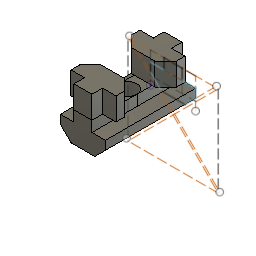
OSSM+Alux (Autodesk Fusion 360 archive; units mm, degrees)
design "4040-t-conector"
Autodesk Fusion 360 part; units mm, degrees
sketch "Sketch1" plane through (0, 0, 0) normal (0, 0, 1) x (1, 0, 0)
  line L0 (20, 0) -> (20, 13.5) construction
  line L1 (20, 13.5) -> (0, 13.5) construction
  line L2 (0, 13.5) -> (0, 0) construction
  line L3 (6, 13.5) -> (14, 13.5)
  line L4 (14, 13.5339) -> (14, 3.75) construction
  line L5 (14, 8.8) -> (6, 8.8) construction
  line L6 (6, 8.8) -> (6, 13.5) construction
  line L7 (0, 3.75) -> (20, 3.75) construction
  line L8 (-10, 13.5339) -> (30, 13.5339) construction
  line L9 (30, 13.5339) -> (30, -26.4661) construction
  line L10 (30, -26.4661) -> (-10, -26.4661) construction
  line L11 (-10, -26.4661) -> (-10, 13.5339) construction
  line L12 (-10, 13.5339) -> (30, -26.4661) construction
  line L13 (-9.2929, 14.241) -> (30.7071, -25.759) construction
  line L14 (30, 13.5339) -> (-10, -26.4661) construction
  line L15 (29.2929, 14.241) -> (-10.7071, -25.759) construction
  line L16 (0, 8.8) -> (20, 8.8) construction
  line L17 (6, 13.5) -> (6, 8.8)
  line L18 (0, 8.8) -> (0, 4.9481)
  line L19 (4.7481, 0.2) -> (15.2519, 0.2)
  line L20 (15.2519, 0.2) -> (20, 4.9481)
  line L21 (20, 4.9481) -> (20, 8.8)
  line L22 (20, 8.8) -> (14, 8.8)
  line L23 (14, 8.8) -> (14, 13.5)
  line L24 (6, 8.8) -> (0, 8.8)
  line L25 (0, 4.9481) -> (4.7481, 0.2)
  dimension "d1" = 20
  dimension "d2" = 13.5
  dimension "d3" = 8
  dimension "d4" = 4.7
  dimension "d5" = 6
  dimension "d6" = 9.75
  dimension "d7" = 40
  dimension "d8" = 40
  dimension "d9" = 10
  dimension "d10" = -1
  dimension "d11" = 1
  dimension "d21" = 13.3
  constraint vertical L0
  constraint horizontal L1
  constraint vertical L2
  constraint coincident L2.end origin
  constraint horizontal L3
  constraint vertical L4
  constraint horizontal L5
  constraint vertical L6
  constraint coincident L1 L3.start
  constraint coincident L2 L7.start
  constraint coincident L0 L7.end
  constraint perpendicular L0 L7
  constraint horizontal L8
  constraint vertical L9
  constraint horizontal L10
  constraint vertical L11
  constraint coincident L2 L16.start
  constraint coincident L0 L16.end
  constraint perpendicular L0 L16
  constraint coincident L13 L18.end
  constraint coincident L2 L18.end
  constraint coincident L13 L19.start
  constraint coincident L15 L19.end
  constraint coincident L15 L20.end
  constraint coincident L0 L20.end
  constraint coincident L7 L4.end
  constraint coincident L5.start L4
  constraint coincident L8 L4.start
  constraint coincident L3.end L4
  measures "d1" distance of L2.end L0.start
  measures "d2" distance of L2.end L1.end
  measures "d3" distance of L3.start L3.end
  measures "d4" distance of L3.start L5.end
  measures "d5" distance of L2 L6
  measures "d6" distance of L1 L7
  measures "d7" distance of L8.start L8.end
  measures "d8" distance of L8.start L10.end
  measures "d9" distance of L2 L11
  measures "d21" distance of L1 L19
extrude "Extrude1" add sketch "Sketch1" along normal blind 40 makes body 1
sketch "Sketch3" plane through (0, 0, 0) normal (0, 0, 1) x (1, 0, 0)
copy_body "CopyPasteBodies2" bodies 1 makes body 2
copy_body "CopyPasteBodies3" bodies 1 makes body 3
move_body "Move3" bodies 3 to x (1, 0, 0) y (0, 0, 1) z (0, -1, 0) at (0, 53.5, 26.5)
copy_body "CopyPasteBodies4" bodies 1 makes body 4
move_body "Move4" bodies 4 to x (1, 0, 0) y (0, 0, -1) z (0, 1, 0) at (0, 13.5, 13.5)
move_face "OffsetFaces1" offset -30 1 faces at (8.6667, 53.5, 29.5667) on bodies 3
move_face "OffsetFaces2" offset -20 1 faces at (8.6667, 53.5, 10.4333) on bodies 4
sketch "Sketch4" plane through (0, 13.5, 0) normal (0, 1, 0) x (-1, 0, 0)
  line L0 (-14, 0) -> (-6, 0)
  line L1 (-6, 0) -> (-6, 40)
  line L2 (-6, 40) -> (-14, 40)
  line L3 (-14, 40) -> (-14, 0)
  circle A0 centre (-10, 20) radius 4
  line L4 (0, 0) -> (0, 40)
  line L5 (-20, 0) -> (-20, 40)
  dimension "d16" = 8
  dimension "d17" = 20
  dimension "d18" = 10
  dimension "d22" = 20
  measures "d16" diameter of A0
  measures "d17" distance of L0 A0.centre
  measures "d18" distance of A0.centre L4
  measures "d22" distance of L4 L5
extrude "Extrude2" cut sketch "Sketch4" against normal blind 17 contours A0 bodies 1 2
combine "Combine1" operation add target body 3 tool bodies 1 4
copy_body "Body->Comp1" bodies 2 removing the originals makes body 5 in component "t-block"
move_face "OffsetFaces3" offset -10 1 faces at (8.6667, 33.5, 10.4333) on bodies 3
component "t-block" placed x (1, 0, 0) y (0, 1, 0) z (0, 0, 1) at (0, 0, 0)
equation "d5 = ( d1 - d3 ) / 2"
equation "d9 = ( d7 - d1 ) / 2"
equation "d18 = d22 / 2"
named bodies: "t-block"

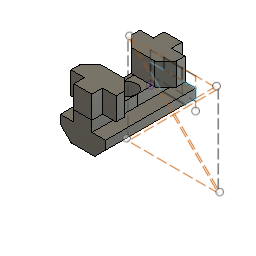
design "4040-t-conector v3"
Autodesk Fusion 360 part; units mm, degrees
sketch "Sketch1" plane through (0, 0, 0) normal (0, 0, 1) x (1, 0, 0)
  line L0 (20, 0) -> (20, 13.5) construction
  line L1 (20, 13.5) -> (0, 13.5) construction
  line L2 (0, 13.5) -> (0, 0) construction
  line L3 (6, 13.5) -> (14, 13.5)
  line L4 (14, 13.5339) -> (14, 3.75) construction
  line L5 (14, 8.8) -> (6, 8.8) construction
  line L6 (6, 8.8) -> (6, 13.5) construction
  line L7 (0, 3.75) -> (20, 3.75) construction
  line L8 (-10, 13.5339) -> (30, 13.5339) construction
  line L9 (30, 13.5339) -> (30, -26.4661) construction
  line L10 (30, -26.4661) -> (-10, -26.4661) construction
  line L11 (-10, -26.4661) -> (-10, 13.5339) construction
  line L12 (-10, 13.5339) -> (30, -26.4661) construction
  line L13 (-9.2929, 14.241) -> (30.7071, -25.759) construction
  line L14 (30, 13.5339) -> (-10, -26.4661) construction
  line L15 (29.2929, 14.241) -> (-10.7071, -25.759) construction
  line L16 (0, 8.8) -> (20, 8.8) construction
  line L17 (6, 13.5) -> (6, 8.8)
  line L18 (0, 8.8) -> (0, 4.9481)
  line L19 (4.7481, 0.2) -> (15.2519, 0.2)
  line L20 (15.2519, 0.2) -> (20, 4.9481)
  line L21 (20, 4.9481) -> (20, 8.8)
  line L22 (20, 8.8) -> (14, 8.8)
  line L23 (14, 8.8) -> (14, 13.5)
  line L24 (6, 8.8) -> (0, 8.8)
  line L25 (0, 4.9481) -> (4.7481, 0.2)
  dimension "d1" = 20
  dimension "d2" = 13.5
  dimension "d3" = 8
  dimension "d4" = 4.7
  dimension "d5" = 6
  dimension "d6" = 9.75
  dimension "d7" = 40
  dimension "d8" = 40
  dimension "d9" = 10
  dimension "d10" = -1
  dimension "d11" = 1
  dimension "d21" = 13.3
  constraint vertical L0
  constraint horizontal L1
  constraint vertical L2
  constraint coincident L2.end origin
  constraint horizontal L3
  constraint vertical L4
  constraint horizontal L5
  constraint vertical L6
  constraint coincident L1 L3.start
  constraint coincident L2 L7.start
  constraint coincident L0 L7.end
  constraint perpendicular L0 L7
  constraint horizontal L8
  constraint vertical L9
  constraint horizontal L10
  constraint vertical L11
  constraint coincident L2 L16.start
  constraint coincident L0 L16.end
  constraint perpendicular L0 L16
  constraint coincident L13 L18.end
  constraint coincident L2 L18.end
  constraint coincident L13 L19.start
  constraint coincident L15 L19.end
  constraint coincident L15 L20.end
  constraint coincident L0 L20.end
  constraint coincident L7 L4.end
  constraint coincident L5.start L4
  constraint coincident L8 L4.start
  constraint coincident L3.end L4
  measures "d1" distance of L2.end L0.start
  measures "d2" distance of L2.end L1.end
  measures "d3" distance of L3.start L3.end
  measures "d4" distance of L3.start L5.end
  measures "d5" distance of L2 L6
  measures "d6" distance of L1 L7
  measures "d7" distance of L8.start L8.end
  measures "d8" distance of L8.start L10.end
  measures "d9" distance of L2 L11
  measures "d21" distance of L1 L19
extrude "Extrude1" add sketch "Sketch1" along normal blind 40 makes body 1
sketch "Sketch3" plane through (0, 0, 0) normal (0, 0, 1) x (1, 0, 0)
copy_body "CopyPasteBodies2" bodies 1 makes body 2
copy_body "CopyPasteBodies3" bodies 1 makes body 3
move_body "Move3" bodies 3 to x (1, 0, 0) y (0, 0, 1) z (0, -1, 0) at (0, 53.5, 26.5)
copy_body "CopyPasteBodies4" bodies 1 makes body 4
move_body "Move4" bodies 4 to x (1, 0, 0) y (0, 0, -1) z (0, 1, 0) at (0, 13.5, 13.5)
move_face "OffsetFaces1" offset -30 1 faces at (8.6667, 53.5, 29.5667) on bodies 3
move_face "OffsetFaces2" offset -20 1 faces at (8.6667, 53.5, 10.4333) on bodies 4
sketch "Sketch4" plane through (0, 13.5, 0) normal (0, 1, 0) x (-1, 0, 0)
  line L0 (-14, 0) -> (-6, 0)
  line L1 (-6, 0) -> (-6, 40)
  line L2 (-6, 40) -> (-14, 40)
  line L3 (-14, 40) -> (-14, 0)
  circle A0 centre (-10, 20) radius 4
  line L4 (0, 0) -> (0, 40)
  line L5 (-20, 0) -> (-20, 40)
  dimension "d16" = 8
  dimension "d17" = 20
  dimension "d18" = 10
  dimension "d22" = 20
  measures "d16" diameter of A0
  measures "d17" distance of L0 A0.centre
  measures "d18" distance of A0.centre L4
  measures "d22" distance of L4 L5
extrude "Extrude2" cut sketch "Sketch4" against normal blind 17 contours A0 bodies 1 2
combine "Combine1" operation add target body 3 tool bodies 1 4
copy_body "Body->Comp1" bodies 2 removing the originals makes body 5 in component "t-block"
move_face "OffsetFaces3" offset -10 1 faces at (8.6667, 33.5, 10.4333) on bodies 3
component "t-block" placed x (1, 0, 0) y (0, 1, 0) z (0, 0, 1) at (0, 0, 0)
equation "d5 = ( d1 - d3 ) / 2"
equation "d9 = ( d7 - d1 ) / 2"
equation "d18 = d22 / 2"
named bodies: "t-block"

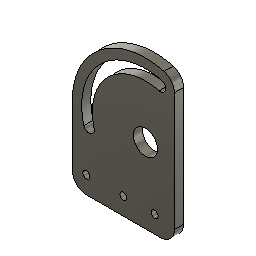
design "hinge-plate v1"
Autodesk Fusion 360 part; units mm, degrees
sketch "Sketch1" plane through (0, 0, 0) normal (0, 0, 1) x (1, 0, 0)
  circle A0 centre (0, 0) radius 10.5
  circle A1 centre (0, 0) radius 4
  arc A2 (11.8123, 44.4575) -> (-44.4575, -11.8123) centre (0, 0) ccw
  arc A3 (14.1876, 53.3973) -> (-53.3973, -14.1876) centre (0, 0) ccw
  arc A4 (-53.3973, -14.1876) -> (-44.4575, -11.8123) centre (-48.9274, -13) ccw
  arc A5 (11.8123, 44.4575) -> (14.1876, 53.3973) centre (13, 48.9274) ccw
  line L0 (25, 58.0996) -> (25, -65)
  line L1 (-63.25, -65) -> (25, -65)
  line L2 (-63.25, 0) -> (-63.25, -65)
  arc A6 (25, 58.0996) -> (-63.25, 0) centre (0, 0) ccw
  circle A7 centre (-51.25, -50) radius 3
  circle A8 centre (-19.125, -50) radius 3
  circle A9 centre (8, -50) radius 3
  dimension "d1" = 21
  dimension "d2" = 8
  dimension "d3" = 92
  dimension "d4" = 110.5
  dimension "d5" = 9.25
  dimension "d6" = 9.25
  dimension "d9" = 126.5
  dimension "d10" = 25
  dimension "d11" = 12
  dimension "d13" = 6
  dimension "d14" = 6
  dimension "d15" = 6
  dimension "d16" = 15
  dimension "d18" = 15
  dimension "d19" = 15
  dimension "d21" = 12
  dimension "d22" = 17
  dimension "d29" = 65
  dimension "d30" = 50.625
  dimension "d33" = 44.125
  dimension "d34" = 13
  constraint coincident A0.centre A1.centre
  constraint concentric A0 A1
  constraint concentric A0 A2
  constraint concentric A0 A3
  constraint concentric A2 A6
  constraint vertical L0
  constraint parallel L0 L2
  constraint tangent L2 A6
  constraint perpendicular L1 L2
  measures "d1" diameter of A0
  measures "d2" diameter of A1
  measures "d3" diameter of A2
  measures "d4" diameter of A3
  measures "d5" diameter of A5
  measures "d6" diameter of A4
  measures "d9" diameter of A6
  measures "d10" distance of A0.centre L0
  measures "d11" distance of A5.centre L0
  measures "d13" diameter of A7
  measures "d14" diameter of A8
  measures "d15" diameter of A9
  measures "d16" distance of L1 A9.centre
  measures "d18" distance of L1 A8.centre
  measures "d19" distance of L1 A7.centre
  measures "d21" distance of L2 A7.centre
  measures "d22" distance of L0 A9.centre
  measures "d29" distance of A0.centre L1
  measures "d30" distance of A0.centre A5.centre
  measures "d33" distance of L0 A8.centre
  measures "d34" vertical distance of A4.centre A0.centre
extrude "Extrude1" add sketch "Sketch1" along normal blind 8 contours L0 L1 L2 A6
fillet "Fillet1" radius 12 3 edges at (-63.25, -65, 4) (25, -65, 4) (25, 58.0996, 4)
equation "d4 = d3 + 18.5 mm"
equation "d5 = d6"
equation "d6 = ( d4 - d3 ) / 2"
equation "d9 = d4 + 16 mm"
equation "d18 = d16"
equation "d19 = d16"
equation "d21 = d11"
equation "d22 = d11 + 5 mm"
equation "d33 = ( ( d9 / 2 ) + d10 ) / 2"
equation "d34 = d10 - d11"
